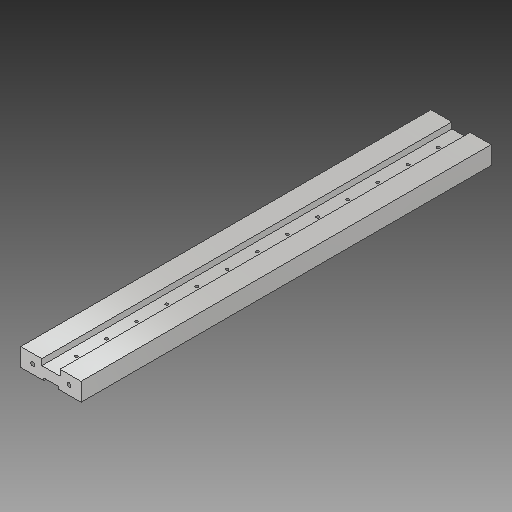
# Autodesk Inventor part: Zcolumn
Saved by Autodesk Inventor 2019 (Build 230136000, 136)
## iProperties
Created: 2018-10-03
Part Number: Zcolumn
Material: Aluminum 6061-AHC
Document SubType Name: Modeling
Designer: LillaHunden
Density: 2.7 g/cm^3
Appearance: Aluminum - Dark
Mass: 595.165 g
Surface Area: 512.389 cm^2
Volume: 220.432 cm^3
Author: LillaHunden
Autodesk Inventor part; units mm, degrees
ref_plane "YZ Plane" through (0, 0, 0) normal (1, 0, 0) x (0, 1, 0)
ref_plane "XZ Plane" through (0, 0, 0) normal (0, 1, 0) x (-1, 0, 0)
ref_plane "XY Plane" through (0, 0, 0) normal (0, 0, 1) x (1, 0, 0)
sketch "Sketch1" plane through (0, 0, 0) normal (0, 0, 1) x (1, 0, 0)
  line L0 (-83.9793, 28.2703) -> (-133.9793, 28.2703)
  line L1 (-133.9793, 28.2703) -> (-133.9793, 43.2703)
  line L2 (-133.9793, 43.2703) -> (-83.9793, 43.2703)
  line L3 (-83.9793, 43.2703) -> (-83.9793, 28.2703)
  point P0 (0, 0)
  dimension "d0" = 50
  dimension "d1" = 15
  constraints: 8 end point, 2 parallel, 1 horizontal, 1 perpendicular
  measures "d0" distance of L1.end L2.end
  measures "d1" distance of L0.end L1.end
extrude "Extrusion1" add sketch "Sketch1" along normal blind 340
sketch "Sketch2" plane through (-133.9793, 43.2703, 0) normal (0, 1, 0) x (1, 0, 0)
  line L0 (50, 0) -> (0, 0) projected
  line L1 (32.55, -340) -> (17.45, -340)
  line L2 (17.45, -340) -> (17.45, 0)
  line L3 (17.45, 0) -> (32.55, 0)
  line L4 (32.55, 0) -> (32.55, -340)
  line L5 (50, -340) -> (0, -340) projected
  point P0 (133.9793, 0)
  point P1 (25, -340)
  dimension "d4" = 15.1
  constraints: 8 end point, 2 midpoint, 2 parallel, 1 horizontal, 1 perpendicular, 1 point on line
  measures "d4" distance between parallel lines of L4 L2
extrude "Extrusion2" cut sketch "Sketch2" against normal blind 5
sketch "Sketch3" plane through (-133.9793, 28.2703, 0) normal (0, -1, 0) x (1, 0, 0)
  line L0 (17.45, 340) -> (0, 340) projected
  line L1 (17.45, 0) -> (32.55, 0) projected
  line L2 (19, 340) -> (31, 340)
  line L3 (31, 340) -> (31, 0)
  line L4 (31, 0) -> (19, 0)
  line L5 (19, 0) -> (19, 340)
  line L6 (0, 340) -> (50, 340) projected
  point P0 (133.9793, 0)
  point P1 (25, 340)
  dimension "d7" = 12
  constraints: 8 end point, 2 midpoint, 2 parallel, 2 point on line, 1 horizontal, 1 perpendicular
  measures "d7" distance of L3.end L4.end
extrude "Extrusion3" cut sketch "Sketch3" against normal blind 2
sketch "Sketch5" plane through (0, 0, 340) normal (0, 0, 1) x (1, 0, 0)
  point P0 (-93.9793, 35.7703)
  point P1 (-123.9793, 35.7703)
hole "Hole2" at (-93.9793, 35.7703, 340) at (-123.9793, 35.7703, 340) direction (0, 0, -1) diameter 3.242 depth 14.5 tip angle 120 thread size "M4x0.7" class "6H" standard "ISO Metric profile"
sketch "Sketch7" plane through (-133.9793, 30.2703, 0) normal (0, -1, 0) x (1, 0, 0)
  point P0 (25, 319)
  point P1 (25, 294)
  point P2 (25, 269)
  point P3 (25, 244)
  point P4 (25, 219)
  point P5 (25, 194)
  point P6 (25, 169)
  point P7 (25, 144)
  point P8 (25, 119)
  point P9 (25, 94)
  point P10 (25, 69)
  point P11 (25, 44)
  point P12 (25, 19)
hole "Hole4" at (-108.9793, 30.2703, 319) at (-108.9793, 30.2703, 294) at (-108.9793, 30.2703, 269) at (-108.9793, 30.2703, 244) at (-108.9793, 30.2703, 219) at (-108.9793, 30.2703, 194) at (-108.9793, 30.2703, 169) at (-108.9793, 30.2703, 144) at (-108.9793, 30.2703, 119) at (-108.9793, 30.2703, 94) at (-108.9793, 30.2703, 69) at (-108.9793, 30.2703, 44) at (-108.9793, 30.2703, 19) direction (0, 1, 0) diameter 2.459 depth 24 tip angle 120 thread size "M3x0.5" class "6H" standard "ISO Metric profile"
body "Solid1"
